Autodesk Fusion 360 part; units mm, degrees
note: some values were not read from the file. Chosen so that the rebuilt part matches the saved one: a direction. Set by a fixed rule: which sketch regions a step uses.
(part 5 of 8)
  spline S19 degree 5 poles (-15.803, -23.1572) (-15.8053, -23.1631) (-15.8097, -23.1748) (-15.8163, -23.1924) (-15.8251, -23.2159) (-15.8359, -23.2453) (-15.8465, -23.2747) (-15.857, -23.304) (-15.8673, -23.3334) (-15.8775, -23.3628) (-15.8876, -23.3922) (-15.8975, -23.4216) (-15.9072, -23.451) (-15.9169, -23.4804) (-15.9263, -23.5098) (-15.9356, -23.5392) (-15.9448, -23.5686) (-15.9538, -23.598) (-15.9626, -23.6275) (-15.9713, -23.6569) (-15.9799, -23.6863) (-15.9882, -23.7157) (-15.9965, -23.7451) (-16.0045, -23.7745) (-16.0124, -23.8039) (-16.0202, -23.8333) (-16.0277, -23.8627) (-16.0352, -23.8921) (-16.0424, -23.9215) (-16.0495, -23.9508) (-16.0564, -23.9802) (-16.0632, -24.0096) (-16.0697, -24.0389) (-16.0761, -24.0683) (-16.0824, -24.0976) (-16.0884, -24.1269) (-16.0943, -24.1562) (-16.1, -24.1855) (-16.1055, -24.2148) (-16.1109, -24.2441) (-16.116, -24.2734) (-16.121, -24.3026) (-16.1258, -24.3319) (-16.1303, -24.3611) (-16.1347, -24.3903) (-16.1389, -24.4195) (-16.1429, -24.4487) (-16.1467, -24.4778) (-16.1503, -24.5069) (-16.1537, -24.536) (-16.1569, -24.5651) (-16.1598, -24.5942) (-16.1625, -24.6232) (-16.165, -24.6522) (-16.1672, -24.6812) (-16.1692, -24.7101) (-16.171, -24.7391) (-16.1726, -24.768) (-16.174, -24.7968) (-16.1751, -24.8257) (-16.1759, -24.8544) (-16.1763, -24.8832) (-16.1764, -24.9118) (-16.1761, -24.9405) (-16.1754, -24.969) (-16.1745, -24.9976) (-16.1735, -25.0261) (-16.1722, -25.0545) (-16.1707, -25.0829) (-16.1687, -25.1112) (-16.1659, -25.1394) (-16.1628, -25.1618) (-16.1599, -25.1785) (-16.1576, -25.1896) (-16.1565, -25.1951) knots -1 -1 -1 -1 -1 -1 -0.98571429 -0.97142857 -0.95714286 -0.94285714 -0.92857143 -0.91428571 -0.9 -0.88571429 -0.87142857 -0.85714286 -0.84285714 -0.82857143 -0.81428571 -0.8 -0.78571429 -0.77142857 -0.75714286 -0.74285714 -0.72857143 -0.71428571 -0.7 -0.68571429 -0.67142857 -0.65714286 -0.64285714 -0.62857143 -0.61428571 -0.6 -0.58571429 -0.57142857 -0.55714286 -0.54285714 -0.52857143 -0.51428571 -0.5 -0.48571429 -0.47142857 -0.45714286 -0.44285714 -0.42857143 -0.41428571 -0.4 -0.38571429 -0.37142857 -0.35714286 -0.34285714 -0.32857143 -0.31428571 -0.3 -0.28571429 -0.27142857 -0.25714286 -0.24285714 -0.22857143 -0.21428571 -0.2 -0.18571429 -0.17142857 -0.15714286 -0.14285714 -0.12857143 -0.11428571 -0.1 -0.08571429 -0.07142857 -0.05714286 -0.04285714 -0.02857143 -0.01428571 0 0 0 0 0 0
  line L19 (-16.1565, -25.1951) -> (-16.0752, -25.5744)
  arc A39 (-16.1513, -25.6929) -> (-16.0752, -25.5744) centre (-16.173, -25.5953) ccw
  arc A40 (-16.1513, -25.6929) -> (-17.1506, -25.9604) centre (-13.5, -37.5997) ccw
  arc A41 (-17.2757, -25.8957) -> (-17.1506, -25.9604) centre (-17.1805, -25.865) ccw
  line L20 (-17.2757, -25.8957) -> (-17.3947, -25.5265)
  spline S20 degree 5 poles (-17.3947, -25.5265) (-17.3965, -25.5211) (-17.4001, -25.5104) (-17.4059, -25.4945) (-17.4144, -25.4735) (-17.426, -25.4477) (-17.4384, -25.4222) (-17.4513, -25.3969) (-17.4645, -25.3716) (-17.4778, -25.3464) (-17.4912, -25.3212) (-17.505, -25.2961) (-17.519, -25.2712) (-17.5334, -25.2464) (-17.5481, -25.2217) (-17.5632, -25.1972) (-17.5785, -25.1727) (-17.5941, -25.1484) (-17.6099, -25.1242) (-17.6259, -25.1) (-17.6421, -25.0759) (-17.6585, -25.052) (-17.6752, -25.0281) (-17.692, -25.0043) (-17.7091, -24.9806) (-17.7263, -24.9569) (-17.7438, -24.9334) (-17.7615, -24.91) (-17.7793, -24.8866) (-17.7974, -24.8634) (-17.8156, -24.8402) (-17.834, -24.817) (-17.8525, -24.794) (-17.8713, -24.7711) (-17.8902, -24.7482) (-17.9093, -24.7254) (-17.9285, -24.7027) (-17.9479, -24.6801) (-17.9675, -24.6576) (-17.9872, -24.6351) (-18.0071, -24.6127) (-18.0272, -24.5904) (-18.0474, -24.5682) (-18.0677, -24.5461) (-18.0883, -24.524) (-18.1089, -24.502) (-18.1297, -24.4801) (-18.1507, -24.4583) (-18.1718, -24.4365) (-18.193, -24.4148) (-18.2144, -24.3932) (-18.236, -24.3717) (-18.2576, -24.3503) (-18.2794, -24.3289) (-18.3014, -24.3076) (-18.3235, -24.2864) (-18.3457, -24.2653) (-18.3681, -24.2442) (-18.3905, -24.2232) (-18.4132, -24.2023) (-18.4359, -24.1815) (-18.4588, -24.1607) (-18.4818, -24.1401) (-18.505, -24.1195) (-18.5282, -24.0989) (-18.5516, -24.0785) (-18.5751, -24.0581) (-18.5988, -24.0378) (-18.6225, -24.0176) (-18.6464, -23.9975) (-18.6704, -23.9774) (-18.6897, -23.9615) (-18.7043, -23.9495) (-18.714, -23.9415) (-18.7189, -23.9376) knots 0 0 0 0 0 0 0.01428571 0.02857143 0.04285714 0.05714286 0.07142857 0.08571429 0.1 0.11428571 0.12857143 0.14285714 0.15714286 0.17142857 0.18571429 0.2 0.21428571 0.22857143 0.24285714 0.25714286 0.27142857 0.28571429 0.3 0.31428571 0.32857143 0.34285714 0.35714286 0.37142857 0.38571429 0.4 0.41428571 0.42857143 0.44285714 0.45714286 0.47142857 0.48571429 0.5 0.51428571 0.52857143 0.54285714 0.55714286 0.57142857 0.58571429 0.6 0.61428571 0.62857143 0.64285714 0.65714286 0.67142857 0.68571429 0.7 0.71428571 0.72857143 0.74285714 0.75714286 0.77142857 0.78571429 0.8 0.81428571 0.82857143 0.84285714 0.85714286 0.87142857 0.88571429 0.9 0.91428571 0.92857143 0.94285714 0.95714286 0.97142857 0.98571429 1 1 1 1 1 1
  arc A42 (-18.7189, -23.9376) -> (-19.4626, -24.2454) centre (-13.5, -37.5997) ccw
  spline S21 degree 5 poles (-19.4626, -24.2454) (-19.4632, -24.2516) (-19.4645, -24.2641) (-19.4663, -24.2828) (-19.4687, -24.3078) (-19.4715, -24.339) (-19.4741, -24.3701) (-19.4767, -24.4012) (-19.4791, -24.4322) (-19.4813, -24.4633) (-19.4834, -24.4943) (-19.4854, -24.5252) (-19.4872, -24.5562) (-19.4888, -24.587) (-19.4904, -24.6179) (-19.4918, -24.6487) (-19.493, -24.6795) (-19.4941, -24.7102) (-19.495, -24.7409) (-19.4958, -24.7716) (-19.4964, -24.8022) (-19.4969, -24.8328) (-19.4972, -24.8633) (-19.4974, -24.8938) (-19.4974, -24.9242) (-19.4973, -24.9546) (-19.497, -24.985) (-19.4966, -25.0153) (-19.496, -25.0456) (-19.4952, -25.0758) (-19.4943, -25.1059) (-19.4932, -25.136) (-19.492, -25.1661) (-19.4906, -25.1961) (-19.489, -25.226) (-19.4873, -25.2559) (-19.4853, -25.2858) (-19.4833, -25.3156) (-19.481, -25.3453) (-19.4786, -25.3749) (-19.476, -25.4045) (-19.4732, -25.4341) (-19.4703, -25.4636) (-19.4671, -25.493) (-19.4638, -25.5223) (-19.4603, -25.5516) (-19.4566, -25.5808) (-19.4527, -25.6099) (-19.4487, -25.639) (-19.4444, -25.668) (-19.4399, -25.6969) (-19.4353, -25.7258) (-19.4304, -25.7545) (-19.4252, -25.7831) (-19.4199, -25.8117) (-19.4143, -25.8402) (-19.4086, -25.8686) (-19.4026, -25.8969) (-19.3965, -25.9252) (-19.3901, -25.9533) (-19.3834, -25.9813) (-19.3764, -26.0092) (-19.369, -26.0369) (-19.3613, -26.0644) (-19.3533, -26.0919) (-19.3451, -26.1192) (-19.3367, -26.1464) (-19.3281, -26.1736) (-19.3193, -26.2006) (-19.31, -26.2275) (-19.3, -26.254) (-19.2912, -26.2748) (-19.2841, -26.2902) (-19.2791, -26.3003) (-19.2765, -26.3053) knots -1 -1 -1 -1 -1 -1 -0.98571429 -0.97142857 -0.95714286 -0.94285714 -0.92857143 -0.91428571 -0.9 -0.88571429 -0.87142857 -0.85714286 -0.84285714 -0.82857143 -0.81428571 -0.8 -0.78571429 -0.77142857 -0.75714286 -0.74285714 -0.72857143 -0.71428571 -0.7 -0.68571429 -0.67142857 -0.65714286 -0.64285714 -0.62857143 -0.61428571 -0.6 -0.58571429 -0.57142857 -0.55714286 -0.54285714 -0.52857143 -0.51428571 -0.5 -0.48571429 -0.47142857 -0.45714286 -0.44285714 -0.42857143 -0.41428571 -0.4 -0.38571429 -0.37142857 -0.35714286 -0.34285714 -0.32857143 -0.31428571 -0.3 -0.28571429 -0.27142857 -0.25714286 -0.24285714 -0.22857143 -0.21428571 -0.2 -0.18571429 -0.17142857 -0.15714286 -0.14285714 -0.12857143 -0.11428571 -0.1 -0.08571429 -0.07142857 -0.05714286 -0.04285714 -0.02857143 -0.01428571 0 0 0 0 0 0
  line L21 (-19.2765, -26.3053) -> (-19.0999, -26.6507)
  arc A43 (-19.1426, -26.7849) -> (-19.0999, -26.6507) centre (-19.1889, -26.6962) ccw
  arc A44 (-19.1426, -26.7849) -> (-20.0387, -27.3018) centre (-13.5, -37.5997) ccw
  arc A45 (-20.1762, -27.2717) -> (-20.0387, -27.3018) centre (-20.0923, -27.2174) ccw
  line L22 (-20.1762, -27.2717) -> (-20.3868, -26.946)
  spline S22 degree 5 poles (-20.3868, -26.946) (-20.3899, -26.9412) (-20.3961, -26.9318) (-20.4059, -26.9179) (-20.4195, -26.8999) (-20.4374, -26.8779) (-20.456, -26.8565) (-20.475, -26.8353) (-20.4942, -26.8143) (-20.5136, -26.7934) (-20.5332, -26.7726) (-20.5529, -26.7519) (-20.5729, -26.7315) (-20.5932, -26.7112) (-20.6138, -26.6912) (-20.6347, -26.6714) (-20.6559, -26.6518) (-20.6772, -26.6323) (-20.6988, -26.613) (-20.7205, -26.5938) (-20.7424, -26.5747) (-20.7644, -26.5558) (-20.7867, -26.537) (-20.8091, -26.5184) (-20.8317, -26.4999) (-20.8545, -26.4816) (-20.8775, -26.4634) (-20.9006, -26.4453) (-20.9239, -26.4274) (-20.9473, -26.4096) (-20.9709, -26.3919) (-20.9947, -26.3743) (-21.0186, -26.3569) (-21.0426, -26.3396) (-21.0668, -26.3224) (-21.0911, -26.3053) (-21.1156, -26.2884) (-21.1402, -26.2715) (-21.1649, -26.2548) (-21.1898, -26.2383) (-21.2148, -26.2218) (-21.24, -26.2054) (-21.2652, -26.1892) (-21.2906, -26.1731) (-21.3162, -26.1571) (-21.3418, -26.1412) (-21.3676, -26.1254) (-21.3935, -26.1097) (-21.4195, -26.0942) (-21.4456, -26.0787) (-21.4719, -26.0634) (-21.4983, -26.0482) (-21.5247, -26.0331) (-21.5513, -26.0181) (-21.578, -26.0032) (-21.6049, -25.9884) (-21.6318, -25.9738) (-21.6588, -25.9592) (-21.686, -25.9448) (-21.7133, -25.9304) (-21.7406, -25.9162) (-21.7681, -25.9021) (-21.7957, -25.8881) (-21.8234, -25.8742) (-21.8511, -25.8604) (-21.879, -25.8467) (-21.907, -25.8331) (-21.9351, -25.8196) (-21.9633, -25.8062) (-21.9916, -25.793) (-22.02, -25.7798) (-22.0428, -25.7694) (-22.0599, -25.7616) (-22.0713, -25.7564) (-22.0771, -25.7538) knots 0 0 0 0 0 0 0.01428571 0.02857143 0.04285714 0.05714286 0.07142857 0.08571429 0.1 0.11428571 0.12857143 0.14285714 0.15714286 0.17142857 0.18571429 0.2 0.21428571 0.22857143 0.24285714 0.25714286 0.27142857 0.28571429 0.3 0.31428571 0.32857143 0.34285714 0.35714286 0.37142857 0.38571429 0.4 0.41428571 0.42857143 0.44285714 0.45714286 0.47142857 0.48571429 0.5 0.51428571 0.52857143 0.54285714 0.55714286 0.57142857 0.58571429 0.6 0.61428571 0.62857143 0.64285714 0.65714286 0.67142857 0.68571429 0.7 0.71428571 0.72857143 0.74285714 0.75714286 0.77142857 0.78571429 0.8 0.81428571 0.82857143 0.84285714 0.85714286 0.87142857 0.88571429 0.9 0.91428571 0.92857143 0.94285714 0.95714286 0.97142857 0.98571429 1 1 1 1 1 1
  arc A46 (-22.0771, -25.7538) -> (-22.7158, -26.2436) centre (-13.5, -37.5997) ccw
  spline S23 degree 5 poles (-22.7158, -26.2436) (-22.7148, -26.2498) (-22.7127, -26.2622) (-22.7097, -26.2808) (-22.7055, -26.3055) (-22.7001, -26.3363) (-22.6947, -26.3671) (-22.689, -26.3978) (-22.6833, -26.4284) (-22.6775, -26.459) (-22.6715, -26.4894) (-22.6653, -26.5199) (-22.6591, -26.5502) (-22.6527, -26.5805) (-22.6462, -26.6107) (-22.6396, -26.6408) (-22.6328, -26.6708) (-22.6259, -26.7008) (-22.6188, -26.7307) (-22.6116, -26.7605) (-22.6043, -26.7903) (-22.5969, -26.8199) (-22.5893, -26.8495) (-22.5816, -26.879) (-22.5737, -26.9084) (-22.5657, -26.9377) (-22.5576, -26.967) (-22.5493, -26.9961) (-22.5409, -27.0252) (-22.5324, -27.0542) (-22.5237, -27.0831) (-22.5148, -27.1119) (-22.5059, -27.1406) (-22.4967, -27.1692) (-22.4875, -27.1977) (-22.478, -27.2262) (-22.4685, -27.2545) (-22.4588, -27.2827) (-22.4489, -27.3108) (-22.4389, -27.3389) (-22.4287, -27.3668) (-22.4184, -27.3946) (-22.4079, -27.4223) (-22.3973, -27.4499) (-22.3865, -27.4774) (-22.3755, -27.5048) (-22.3644, -27.532) (-22.3531, -27.5592) (-22.3416, -27.5862) (-22.33, -27.6131) (-22.3182, -27.6399) (-22.3062, -27.6665) (-22.2941, -27.693) (-22.2817, -27.7194) (-22.2691, -27.7456) (-22.2564, -27.7716) (-22.2435, -27.7976) (-22.2304, -27.8234) (-22.2172, -27.8491) (-22.2037, -27.8746) (-22.19, -27.8999) (-22.176, -27.925) (-22.1617, -27.9499) (-22.1472, -27.9745) (-22.1323, -27.9989) (-22.1173, -28.0232) (-22.1021, -28.0473) (-22.0868, -28.0714) (-22.0713, -28.0952) (-22.0554, -28.1187) (-22.0389, -28.1417) (-22.025, -28.1596) (-22.0141, -28.1726) (-22.0066, -28.181) (-22.0029, -28.1852) knots -1 -1 -1 -1 -1 -1 -0.98571429 -0.97142857 -0.95714286 -0.94285714 -0.92857143 -0.91428571 -0.9 -0.88571429 -0.87142857 -0.85714286 -0.84285714 -0.82857143 -0.81428571 -0.8 -0.78571429 -0.77142857 -0.75714286 -0.74285714 -0.72857143 -0.71428571 -0.7 -0.68571429 -0.67142857 -0.65714286 -0.64285714 -0.62857143 -0.61428571 -0.6 -0.58571429 -0.57142857 -0.55714286 -0.54285714 -0.52857143 -0.51428571 -0.5 -0.48571429 -0.47142857 -0.45714286 -0.44285714 -0.42857143 -0.41428571 -0.4 -0.38571429 -0.37142857 -0.35714286 -0.34285714 -0.32857143 -0.31428571 -0.3 -0.28571429 -0.27142857 -0.25714286 -0.24285714 -0.22857143 -0.21428571 -0.2 -0.18571429 -0.17142857 -0.15714286 -0.14285714 -0.12857143 -0.11428571 -0.1 -0.08571429 -0.07142857 -0.05714286 -0.04285714 -0.02857143 -0.01428571 0 0 0 0 0 0
  line L23 (-22.0029, -28.1852) -> (-21.7429, -28.4731)
  arc A47 (-21.7495, -28.6138) -> (-21.7429, -28.4731) centre (-21.8171, -28.5401) ccw
  arc A48 (-21.7495, -28.6138) -> (-22.4811, -29.3451) centre (-13.5, -37.5997) ccw
  arc A49 (-22.6218, -29.3516) -> (-22.4811, -29.3451) centre (-22.5548, -29.2774) ccw
  line L24 (-22.6218, -29.3516) -> (-22.9095, -29.0914)
  spline S24 degree 5 poles (-22.9095, -29.0914) (-22.9137, -29.0876) (-22.9222, -29.0801) (-22.9352, -29.0692) (-22.953, -29.0553) (-22.976, -29.0388) (-22.9995, -29.0229) (-23.0234, -29.0074) (-23.0474, -28.9921) (-23.0715, -28.9769) (-23.0958, -28.9618) (-23.1202, -28.947) (-23.1448, -28.9324) (-23.1697, -28.9181) (-23.1948, -28.9041) (-23.2201, -28.8904) (-23.2456, -28.8769) (-23.2713, -28.8636) (-23.2971, -28.8505) (-23.323, -28.8376) (-23.3491, -28.8249) (-23.3753, -28.8123) (-23.4016, -28.7999) (-23.4281, -28.7877) (-23.4547, -28.7757) (-23.4815, -28.7639) (-23.5084, -28.7523) (-23.5354, -28.7408) (-23.5626, -28.7295) (-23.5898, -28.7184) (-23.6172, -28.7074) (-23.6446, -28.6966) (-23.6722, -28.6859) (-23.6999, -28.6754) (-23.7277, -28.6651) (-23.7557, -28.6549) (-23.7837, -28.6449) (-23.8118, -28.635) (-23.84, -28.6252) (-23.8684, -28.6157) (-23.8968, -28.6062) (-23.9253, -28.5969) (-23.9539, -28.5878) (-23.9826, -28.5788) (-24.0114, -28.5699) (-24.0403, -28.5612) (-24.0693, -28.5527) (-24.0983, -28.5442) (-24.1275, -28.5359) (-24.1567, -28.5278) (-24.1861, -28.5198) (-24.2155, -28.5119) (-24.245, -28.5042) (-24.2745, -28.4966) (-24.3042, -28.4891) (-24.3339, -28.4818) (-24.3637, -28.4746) (-24.3936, -28.4675) (-24.4236, -28.4606) (-24.4536, -28.4538) (-24.4837, -28.4472) (-24.5139, -28.4406) (-24.5442, -28.4342) (-24.5745, -28.428) (-24.605, -28.4218) (-24.6354, -28.4158) (-24.666, -28.4099) (-24.6966, -28.4042) (-24.7273, -28.3986) (-24.758, -28.3931) (-24.7889, -28.3877) (-24.8136, -28.3835) (-24.8321, -28.3804) (-24.8445, -28.3784) (-24.8507, -28.3774) knots 0 0 0 0 0 0 0.01428571 0.02857143 0.04285714 0.05714286 0.07142857 0.08571429 0.1 0.11428571 0.12857143 0.14285714 0.15714286 0.17142857 0.18571429 0.2 0.21428571 0.22857143 0.24285714 0.25714286 0.27142857 0.28571429 0.3 0.31428571 0.32857143 0.34285714 0.35714286 0.37142857 0.38571429 0.4 0.41428571 0.42857143 0.44285714 0.45714286 0.47142857 0.48571429 0.5 0.51428571 0.52857143 0.54285714 0.55714286 0.57142857 0.58571429 0.6 0.61428571 0.62857143 0.64285714 0.65714286 0.67142857 0.68571429 0.7 0.71428571 0.72857143 0.74285714 0.75714286 0.77142857 0.78571429 0.8 0.81428571 0.82857143 0.84285714 0.85714286 0.87142857 0.88571429 0.9 0.91428571 0.92857143 0.94285714 0.95714286 0.97142857 0.98571429 1 1 1 1 1 1
  arc A50 (-24.8507, -28.3774) -> (-25.3409, -29.0158) centre (-13.5, -37.5997) ccw
  spline S25 degree 5 poles (-25.3409, -29.0158) (-25.3383, -29.0215) (-25.3332, -29.033) (-25.3254, -29.0501) (-25.315, -29.0729) (-25.3018, -29.1013) (-25.2886, -29.1296) (-25.2752, -29.1578) (-25.2617, -29.1859) (-25.2482, -29.2139) (-25.2345, -29.2418) (-25.2207, -29.2696) (-25.2068, -29.2973) (-25.1928, -29.3248) (-25.1787, -29.3523) (-25.1645, -29.3797) (-25.1502, -29.407) (-25.1358, -29.4341) (-25.1212, -29.4612) (-25.1066, -29.4881) (-25.0918, -29.515) (-25.0769, -29.5417) (-25.062, -29.5683) (-25.0469, -29.5948) (-25.0317, -29.6211) (-25.0164, -29.6474) (-25.0009, -29.6736) (-24.9854, -29.6996) (-24.9698, -29.7255) (-24.954, -29.7513) (-24.9381, -29.7769) (-24.9221, -29.8025) (-24.906, -29.8279) (-24.8898, -29.8531) (-24.8735, -29.8783) (-24.857, -29.9033) (-24.8404, -29.9282) (-24.8237, -29.953) (-24.8069, -29.9776) (-24.79, -30.0021) (-24.773, -30.0264) (-24.7558, -30.0506) (-24.7385, -30.0746) (-24.7211, -30.0985) (-24.7035, -30.1223) (-24.6858, -30.1459) (-24.668, -30.1693) (-24.6501, -30.1926) (-24.632, -30.2158) (-24.6139, -30.2388) (-24.5955, -30.2616) (-24.5771, -30.2842) (-24.5585, -30.3066) (-24.5397, -30.3289) (-24.5208, -30.351) (-24.5017, -30.3728) (-24.4825, -30.3946) (-24.4632, -30.4161) (-24.4438, -30.4375) (-24.4242, -30.4587) (-24.4044, -30.4796) (-24.3844, -30.5002) (-24.3642, -30.5205) (-24.3437, -30.5405) (-24.323, -30.5603) (-24.3022, -30.5798) (-24.2813, -30.5992) (-24.2603, -30.6185) (-24.2392, -30.6375) (-24.2178, -30.6561) (-24.1959, -30.674) (-24.1778, -30.6877) (-24.1639, -30.6974) (-24.1545, -30.7037) (-24.1498, -30.7067) knots -1 -1 -1 -1 -1 -1 -0.98571429 -0.97142857 -0.95714286 -0.94285714 -0.92857143 -0.91428571 -0.9 -0.88571429 -0.87142857 -0.85714286 -0.84285714 -0.82857143 -0.81428571 -0.8 -0.78571429 -0.77142857 -0.75714286 -0.74285714 -0.72857143 -0.71428571 -0.7 -0.68571429 -0.67142857 -0.65714286 -0.64285714 -0.62857143 -0.61428571 -0.6 -0.58571429 -0.57142857 -0.55714286 -0.54285714 -0.52857143 -0.51428571 -0.5 -0.48571429 -0.47142857 -0.45714286 -0.44285714 -0.42857143 -0.41428571 -0.4 -0.38571429 -0.37142857 -0.35714286 -0.34285714 -0.32857143 -0.31428571 -0.3 -0.28571429 -0.27142857 -0.25714286 -0.24285714 -0.22857143 -0.21428571 -0.2 -0.18571429 -0.17142857 -0.15714286 -0.14285714 -0.12857143 -0.11428571 -0.1 -0.08571429 -0.07142857 -0.05714286 -0.04285714 -0.02857143 -0.01428571 0 0 0 0 0 0
  line L25 (-24.1498, -30.7067) -> (-23.8241, -30.9175)
  arc A51 (-23.7941, -31.0551) -> (-23.8241, -30.9175) centre (-23.8785, -31.0014) ccw
  arc A52 (-23.7941, -31.0551) -> (-24.3116, -31.9508) centre (-13.5, -37.5997) ccw
  arc A53 (-24.4458, -31.9935) -> (-24.3116, -31.9508) centre (-24.4002, -31.9045) ccw
  line L26 (-24.4458, -31.9935) -> (-24.791, -31.8167)
  spline S26 degree 5 poles (-24.791, -31.8167) (-24.7961, -31.8141) (-24.8062, -31.8091) (-24.8216, -31.8019) (-24.8424, -31.7931) (-24.8689, -31.7831) (-24.8957, -31.7738) (-24.9227, -31.765) (-24.9499, -31.7564) (-24.9771, -31.748) (-25.0045, -31.7397) (-25.0319, -31.7317) (-25.0594, -31.724) (-25.0871, -31.7166) (-25.115, -31.7096) (-25.143, -31.7029) (-25.1711, -31.6965) (-25.1994, -31.6903) (-25.2277, -31.6843) (-25.2561, -31.6786) (-25.2846, -31.673) (-25.3131, -31.6676) (-25.3418, -31.6625) (-25.3705, -31.6576) (-25.3993, -31.6529) (-25.4283, -31.6484) (-25.4573, -31.6441) (-25.4863, -31.64) (-25.5155, -31.6361) (-25.5447, -31.6324) (-25.5739, -31.6289) (-25.6033, -31.6256) (-25.6327, -31.6224) (-25.6622, -31.6194) (-25.6917, -31.6166) (-25.7213, -31.614) (-25.751, -31.6116) (-25.7807, -31.6093) (-25.8105, -31.6072) (-25.8403, -31.6053) (-25.8702, -31.6036) (-25.9002, -31.602) (-25.9302, -31.6005) (-25.9602, -31.5993) (-25.9903, -31.5982) (-26.0205, -31.5972) (-26.0507, -31.5965) (-26.0809, -31.5958) (-26.1112, -31.5954) (-26.1416, -31.5951) (-26.172, -31.5949) (-26.2024, -31.5949) (-26.2329, -31.5951) (-26.2635, -31.5954) (-26.294, -31.5959) (-26.3247, -31.5965) (-26.3553, -31.5973) (-26.386, -31.5982) (-26.4167, -31.5992) (-26.4475, -31.6005) (-26.4783, -31.6018) (-26.5092, -31.6033) (-26.5401, -31.605) (-26.571, -31.6068) (-26.602, -31.6087) (-26.633, -31.6108) (-26.664, -31.613) (-26.6951, -31.6154) (-26.7262, -31.6179) (-26.7573, -31.6206) (-26.7885, -31.6234) (-26.8134, -31.6257) (-26.8321, -31.6275) (-26.8446, -31.6288) (-26.8509, -31.6294) knots 0 0 0 0 0 0 0.01428571 0.02857143 0.04285714 0.05714286 0.07142857 0.08571429 0.1 0.11428571 0.12857143 0.14285714 0.15714286 0.17142857 0.18571429 0.2 0.21428571 0.22857143 0.24285714 0.25714286 0.27142857 0.28571429 0.3 0.31428571 0.32857143 0.34285714 0.35714286 0.37142857 0.38571429 0.4 0.41428571 0.42857143 0.44285714 0.45714286 0.47142857 0.48571429 0.5 0.51428571 0.52857143 0.54285714 0.55714286 0.57142857 0.58571429 0.6 0.61428571 0.62857143 0.64285714 0.65714286 0.67142857 0.68571429 0.7 0.71428571 0.72857143 0.74285714 0.75714286 0.77142857 0.78571429 0.8 0.81428571 0.82857143 0.84285714 0.85714286 0.87142857 0.88571429 0.9 0.91428571 0.92857143 0.94285714 0.95714286 0.97142857 0.98571429 1 1 1 1 1 1
  arc A54 (-26.8509, -31.6294) -> (-27.1591, -32.3729) centre (-13.5, -37.5997) ccw
  spline S27 degree 5 poles (-27.1591, -32.3729) (-27.1551, -32.3778) (-27.1472, -32.3875) (-27.1353, -32.4021) (-27.1193, -32.4214) (-27.0992, -32.4454) (-27.0791, -32.4693) (-27.0589, -32.4931) (-27.0386, -32.5167) (-27.0183, -32.5403) (-26.9979, -32.5637) (-26.9773, -32.587) (-26.9568, -32.6101) (-26.9361, -32.6331) (-26.9154, -32.656) (-26.8945, -32.6788) (-26.8737, -32.7014) (-26.8527, -32.7239) (-26.8316, -32.7463) (-26.8105, -32.7685) (-26.7893, -32.7906) (-26.768, -32.8126) (-26.7467, -32.8344) (-26.7253, -32.8561) (-26.7037, -32.8776) (-26.6822, -32.899) (-26.6605, -32.9203) (-26.6388, -32.9414) (-26.6169, -32.9624) (-26.595, -32.9832) (-26.5731, -33.0039) (-26.551, -33.0244) (-26.5289, -33.0448) (-26.5067, -33.065) (-26.4844, -33.0851) (-26.462, -33.105) (-26.4395, -33.1247) (-26.417, -33.1443) (-26.3944, -33.1637) (-26.3717, -33.183) (-26.349, -33.2021) (-26.3261, -33.221) (-26.3032, -33.2398) (-26.2802, -33.2584) (-26.2571, -33.2768) (-26.2339, -33.295) (-26.2106, -33.313) (-26.1873, -33.3309) (-26.1638, -33.3486) (-26.1403, -33.3661) (-26.1167, -33.3833) (-26.093, -33.4004) (-26.0692, -33.4173) (-26.0453, -33.4339) (-26.0214, -33.4503) (-25.9973, -33.4665) (-25.9732, -33.4826) (-25.9489, -33.4984) (-25.9246, -33.514) (-25.9002, -33.5294) (-25.8757, -33.5445) (-25.851, -33.5592) (-25.8262, -33.5736) (-25.8013, -33.5876) (-25.7762, -33.6014) (-25.751, -33.6148) (-25.7258, -33.6282) (-25.7006, -33.6413) (-25.6752, -33.6542) (-25.6497, -33.6666) (-25.6239, -33.6783) (-25.603, -33.6868) (-25.587, -33.6926) (-25.5763, -33.6962) (-25.5709, -33.698) knots -1 -1 -1 -1 -1 -1 -0.98571429 -0.97142857 -0.95714286 -0.94285714 -0.92857143 -0.91428571 -0.9 -0.88571429 -0.87142857 -0.85714286 -0.84285714 -0.82857143 -0.81428571 -0.8 -0.78571429 -0.77142857 -0.75714286 -0.74285714 -0.72857143 -0.71428571 -0.7 -0.68571429 -0.67142857 -0.65714286 -0.64285714 -0.62857143 -0.61428571 -0.6 -0.58571429 -0.57142857 -0.55714286 -0.54285714 -0.52857143 -0.51428571 -0.5 -0.48571429 -0.47142857 -0.45714286 -0.44285714 -0.42857143 -0.41428571 -0.4 -0.38571429 -0.37142857 -0.35714286 -0.34285714 -0.32857143 -0.31428571 -0.3 -0.28571429 -0.27142857 -0.25714286 -0.24285714 -0.22857143 -0.21428571 -0.2 -0.18571429 -0.17142857 -0.15714286 -0.14285714 -0.12857143 -0.11428571 -0.1 -0.08571429 -0.07142857 -0.05714286 -0.04285714 -0.02857143 -0.01428571 0 0 0 0 0 0
  line L27 (-25.5709, -33.698) -> (-25.2018, -33.8173)
  arc A55 (-25.1372, -33.9424) -> (-25.2018, -33.8173) centre (-25.2326, -33.9124) ccw
  arc A56 (-25.1372, -33.9424) -> (-25.4052, -34.9415) centre (-13.5, -37.5997) ccw
  arc A57 (-25.5238, -35.0175) -> (-25.4052, -34.9415) centre (-25.5028, -34.9197) ccw
  line L28 (-25.5238, -35.0175) -> (-25.9031, -34.9361)
  spline S28 degree 5 poles (-25.9031, -34.9361) (-25.9086, -34.9349) (-25.9197, -34.9327) (-25.9364, -34.9297) (-25.9588, -34.9266) (-25.9869, -34.9238) (-26.0153, -34.9218) (-26.0437, -34.9202) (-26.0721, -34.919) (-26.1006, -34.9179) (-26.1291, -34.917) (-26.1577, -34.9163) (-26.1863, -34.916) (-26.215, -34.916) (-26.2437, -34.9164) (-26.2725, -34.9172) (-26.3013, -34.9183) (-26.3302, -34.9197) (-26.3591, -34.9212) (-26.388, -34.923) (-26.417, -34.925) (-26.4459, -34.9272) (-26.4749, -34.9297) (-26.504, -34.9324) (-26.533, -34.9353) (-26.5621, -34.9384) (-26.5912, -34.9418) (-26.6204, -34.9454) (-26.6495, -34.9492) (-26.6787, -34.9532) (-26.7079, -34.9573) (-26.7371, -34.9617) (-26.7663, -34.9663) (-26.7956, -34.971) (-26.8248, -34.976) (-26.8541, -34.9811) (-26.8834, -34.9864) (-26.9127, -34.9919) (-26.942, -34.9976) (-26.9713, -35.0035) (-27.0006, -35.0095) (-27.03, -35.0157) (-27.0593, -35.0221) (-27.0887, -35.0287) (-27.118, -35.0354) (-27.1474, -35.0423) (-27.1768, -35.0494) (-27.2062, -35.0566) (-27.2356, -35.064) (-27.265, -35.0716) (-27.2944, -35.0793) (-27.3238, -35.0872) (-27.3532, -35.0952) (-27.3826, -35.1034) (-27.412, -35.1118) (-27.4414, -35.1203) (-27.4708, -35.129) (-27.5002, -35.1378) (-27.5297, -35.1468) (-27.5591, -35.1559) (-27.5885, -35.1652) (-27.6179, -35.1747) (-27.6473, -35.1843) (-27.6767, -35.194) (-27.7061, -35.2039) (-27.7355, -35.2139) (-27.7649, -35.2241) (-27.7943, -35.2344) (-27.8237, -35.2449) (-27.8531, -35.2555) (-27.8825, -35.2663) (-27.906, -35.275) (-27.9236, -35.2816) (-27.9353, -35.2861) (-27.9412, -35.2883) knots 0 0 0 0 0 0 0.01428571 0.02857143 0.04285714 0.05714286 0.07142857 0.08571429 0.1 0.11428571 0.12857143 0.14285714 0.15714286 0.17142857 0.18571429 0.2 0.21428571 0.22857143 0.24285714 0.25714286 0.27142857 0.28571429 0.3 0.31428571 0.32857143 0.34285714 0.35714286 0.37142857 0.38571429 0.4 0.41428571 0.42857143 0.44285714 0.45714286 0.47142857 0.48571429 0.5 0.51428571 0.52857143 0.54285714 0.55714286 0.57142857 0.58571429 0.6 0.61428571 0.62857143 0.64285714 0.65714286 0.67142857 0.68571429 0.7 0.71428571 0.72857143 0.74285714 0.75714286 0.77142857 0.78571429 0.8 0.81428571 0.82857143 0.84285714 0.85714286 0.87142857 0.88571429 0.9 0.91428571 0.92857143 0.94285714 0.95714286 0.97142857 0.98571429 1 1 1 1 1 1
  arc A58 (-27.9412, -35.2883) -> (-28.0465, -36.0863) centre (-13.5, -37.5997) ccw
  spline S29 degree 5 poles (-28.0465, -36.0863) (-28.0414, -36.09) (-28.0312, -36.0973) (-28.0159, -36.1082) (-27.9955, -36.1228) (-27.9699, -36.1408) (-27.9443, -36.1587) (-27.9186, -36.1764) (-27.8929, -36.194) (-27.8671, -36.2115) (-27.8413, -36.2288) (-27.8155, -36.246) (-27.7896, -36.263) (-27.7637, -36.2799) (-27.7378, -36.2966) (-27.7118, -36.3132) (-27.6857, -36.3297) (-27.6597, -36.346) (-27.6335, -36.3621) (-27.6074, -36.3782) (-27.5812, -36.394) (-27.5549, -36.4097) (-27.5287, -36.4253) (-27.5024, -36.4407) (-27.476, -36.4559) (-27.4496, -36.471) (-27.4232, -36.4859) (-27.3967, -36.5007) (-27.3702, -36.5153) (-27.3437, -36.5298) (-27.3171, -36.544) (-27.2905, -36.5582) (-27.2638, -36.5721) (-27.2371, -36.5859) (-27.2104, -36.5995) (-27.1837, -36.6129) (-27.1569, -36.6262) (-27.13, -36.6393) (-27.1032, -36.6522) (-27.0763, -36.6649) (-27.0493, -36.6775) (-27.0224, -36.6899) (-26.9953, -36.702) (-26.9683, -36.714) (-26.9412, -36.7258) (-26.9141, -36.7374) (-26.887, -36.7488) (-26.8598, -36.76) (-26.8326, -36.7711) (-26.8054, -36.7819) (-26.7781, -36.7925) (-26.7508, -36.8028) (-26.7234, -36.8129) (-26.6961, -36.8228) (-26.6687, -36.8325) (-26.6412, -36.8419) (-26.6137, -36.8511) (-26.5862, -36.8602) (-26.5587, -36.869) (-26.5312, -36.8775) (-26.5036, -36.8857) (-26.4759, -36.8936) (-26.4482, -36.901) (-26.4205, -36.9081) (-26.3927, -36.9149) (-26.365, -36.9214) (-26.3372, -36.9278) (-26.3094, -36.9339) (-26.2815, -36.9398) (-26.2537, -36.9452) (-26.2257, -36.9498) (-26.2033, -36.9526) (-26.1864, -36.9541) (-26.1751, -36.9548) (-26.1695, -36.9551) knots -1 -1 -1 -1 -1 -1 -0.98571429 -0.97142857 -0.95714286 -0.94285714 -0.92857143 -0.91428571 -0.9 -0.88571429 -0.87142857 -0.85714286 -0.84285714 -0.82857143 -0.81428571 -0.8 -0.78571429 -0.77142857 -0.75714286 -0.74285714 -0.72857143 -0.71428571 -0.7 -0.68571429 -0.67142857 -0.65714286 -0.64285714 -0.62857143 -0.61428571 -0.6 -0.58571429 -0.57142857 -0.55714286 -0.54285714 -0.52857143 -0.51428571 -0.5 -0.48571429 -0.47142857 -0.45714286 -0.44285714 -0.42857143 -0.41428571 -0.4 -0.38571429 -0.37142857 -0.35714286 -0.34285714 -0.32857143 -0.31428571 -0.3 -0.28571429 -0.27142857 -0.25714286 -0.24285714 -0.22857143 -0.21428571 -0.2 -0.18571429 -0.17142857 -0.15714286 -0.14285714 -0.12857143 -0.11428571 -0.1 -0.08571429 -0.07142857 -0.05714286 -0.04285714 -0.02857143 -0.01428571 0 0 0 0 0 0
  line L29 (-26.1695, -36.9551) -> (-25.7821, -36.9748)
  arc A59 (-25.6873, -37.079) -> (-25.7821, -36.9748) centre (-25.7872, -37.0747) ccw
  arc A60 (-25.6873, -37.079) -> (-25.6876, -38.1134) centre (-13.5, -37.5997) ccw
  arc A61 (-25.7824, -38.2175) -> (-25.6876, -38.1134) centre (-25.7875, -38.1176) ccw
  line L30 (-25.7824, -38.2175) -> (-26.1698, -38.237)
  spline S30 degree 5 poles (-26.1698, -38.237) (-26.1755, -38.2373) (-26.1868, -38.238) (-26.2037, -38.2395) (-26.2261, -38.2422) (-26.254, -38.2468) (-26.2819, -38.2522) (-26.3097, -38.2581) (-26.3375, -38.2642) (-26.3653, -38.2705) (-26.3931, -38.2771) (-26.4209, -38.2838) (-26.4486, -38.2909) (-26.4763, -38.2984) (-26.504, -38.3062) (-26.5316, -38.3144) (-26.5591, -38.3229) (-26.5867, -38.3317) (-26.6142, -38.3407) (-26.6416, -38.3499) (-26.6691, -38.3593) (-26.6965, -38.369) (-26.7239, -38.3788) (-26.7512, -38.3889) (-26.7786, -38.3993) (-26.8058, -38.4098) (-26.8331, -38.4206) (-26.8603, -38.4316) (-26.8875, -38.4428) (-26.9146, -38.4542) (-26.9417, -38.4658) (-26.9688, -38.4776) (-26.9959, -38.4896) (-27.0229, -38.5017) (-27.0499, -38.5141) (-27.0768, -38.5266) (-27.1037, -38.5393) (-27.1306, -38.5522) (-27.1574, -38.5653) (-27.1842, -38.5786) (-27.211, -38.592) (-27.2377, -38.6056) (-27.2644, -38.6194) (-27.2911, -38.6333) (-27.3177, -38.6474) (-27.3443, -38.6617) (-27.3708, -38.6761) (-27.3974, -38.6907) (-27.4238, -38.7054) (-27.4503, -38.7204) (-27.4767, -38.7354) (-27.503, -38.7507) (-27.5293, -38.766) (-27.5556, -38.7816) (-27.5819, -38.7973) (-27.6081, -38.8131) (-27.6343, -38.8291) (-27.6604, -38.8452) (-27.6865, -38.8615) (-27.7125, -38.878) (-27.7385, -38.8946) (-27.7645, -38.9113) (-27.7904, -38.9282) (-27.8163, -38.9452) (-27.8421, -38.9623) (-27.8679, -38.9797) (-27.8937, -38.9971) (-27.9194, -39.0147) (-27.9451, -39.0324) (-27.9707, -39.0503) (-27.9963, -39.0683) (-28.0168, -39.0828) (-28.0321, -39.0937) (-28.0423, -39.1011) (-28.0474, -39.1047) knots 0 0 0 0 0 0 0.01428571 0.02857143 0.04285714 0.05714286 0.07142857 0.08571429 0.1 0.11428571 0.12857143 0.14285714 0.15714286 0.17142857 0.18571429 0.2 0.21428571 0.22857143 0.24285714 0.25714286 0.27142857 0.28571429 0.3 0.31428571 0.32857143 0.34285714 0.35714286 0.37142857 0.38571429 0.4 0.41428571 0.42857143 0.44285714 0.45714286 0.47142857 0.48571429 0.5 0.51428571 0.52857143 0.54285714 0.55714286 0.57142857 0.58571429 0.6 0.61428571 0.62857143 0.64285714 0.65714286 0.67142857 0.68571429 0.7 0.71428571 0.72857143 0.74285714 0.75714286 0.77142857 0.78571429 0.8 0.81428571 0.82857143 0.84285714 0.85714286 0.87142857 0.88571429 0.9 0.91428571 0.92857143 0.94285714 0.95714286 0.97142857 0.98571429 1 1 1 1 1 1
  arc A62 (-28.0474, -39.1047) -> (-27.9425, -39.9028) centre (-13.5, -37.5997) ccw
  spline S31 degree 5 poles (-27.9425, -39.9028) (-27.9367, -39.905) (-27.9249, -39.9094) (-27.9073, -39.916) (-27.8838, -39.9248) (-27.8544, -39.9356) (-27.8251, -39.9462) (-27.7957, -39.9567) (-27.7663, -39.967) (-27.7369, -39.9772) (-27.7075, -39.9873) (-27.6781, -39.9972) (-27.6487, -40.007) (-27.6193, -40.0166) (-27.5899, -40.026) (-27.5605, -40.0353) (-27.5311, -40.0445) (-27.5017, -40.0535) (-27.4723, -40.0623) (-27.4428, -40.071) (-27.4134, -40.0796) (-27.384, -40.088) (-27.3546, -40.0962) (-27.3252, -40.1042) (-27.2958, -40.1121) (-27.2664, -40.1199) (-27.237, -40.1275) (-27.2076, -40.1349) (-27.1783, -40.1421) (-27.1489, -40.1492) (-27.1195, -40.1561) (-27.0902, -40.1629) (-27.0608, -40.1695) (-27.0315, -40.1759) (-27.0021, -40.1821) (-26.9728, -40.1881) (-26.9435, -40.194) (-26.9142, -40.1997) (-26.8849, -40.2053) (-26.8556, -40.2106) (-26.8263, -40.2157) (-26.7971, -40.2207) (-26.7678, -40.2255) (-26.7386, -40.2301) (-26.7094, -40.2344) (-26.6802, -40.2386) (-26.6511, -40.2426) (-26.6219, -40.2464) (-26.5928, -40.25) (-26.5637, -40.2534) (-26.5346, -40.2566) (-26.5055, -40.2595) (-26.4765, -40.2622) (-26.4475, -40.2647) (-26.4185, -40.2669) (-26.3896, -40.2689) (-26.3606, -40.2707) (-26.3318, -40.2723) (-26.3029, -40.2737) (-26.2741, -40.2748) (-26.2453, -40.2756) (-26.2165, -40.276) (-26.1879, -40.2761) (-26.1592, -40.2758) (-26.1307, -40.2751) (-26.1021, -40.2742) (-26.0737, -40.2732) (-26.0452, -40.2719) (-26.0168, -40.2704) (-25.9885, -40.2684) (-25.9603, -40.2656) (-25.9379, -40.2625) (-25.9212, -40.2596) (-25.9101, -40.2574) (-25.9046, -40.2562) knots -1 -1 -1 -1 -1 -1 -0.98571429 -0.97142857 -0.95714286 -0.94285714 -0.92857143 -0.91428571 -0.9 -0.88571429 -0.87142857 -0.85714286 -0.84285714 -0.82857143 -0.81428571 -0.8 -0.78571429 -0.77142857 -0.75714286 -0.74285714 -0.72857143 -0.71428571 -0.7 -0.68571429 -0.67142857 -0.65714286 -0.64285714 -0.62857143 -0.61428571 -0.6 -0.58571429 -0.57142857 -0.55714286 -0.54285714 -0.52857143 -0.51428571 -0.5 -0.48571429 -0.47142857 -0.45714286 -0.44285714 -0.42857143 -0.41428571 -0.4 -0.38571429 -0.37142857 -0.35714286 -0.34285714 -0.32857143 -0.31428571 -0.3 -0.28571429 -0.27142857 -0.25714286 -0.24285714 -0.22857143 -0.21428571 -0.2 -0.18571429 -0.17142857 -0.15714286 -0.14285714 -0.12857143 -0.11428571 -0.1 -0.08571429 -0.07142857 -0.05714286 -0.04285714 -0.02857143 -0.01428571 0 0 0 0 0 0
  line L31 (-25.9046, -40.2562) -> (-25.5253, -40.1749)
  arc A63 (-25.4068, -40.251) -> (-25.5253, -40.1749) centre (-25.5044, -40.2727) ccw
  arc A64 (-25.4068, -40.251) -> (-25.1393, -41.2503) centre (-13.5, -37.5997) ccw
  arc A65 (-25.204, -41.3754) -> (-25.1393, -41.2503) centre (-25.2347, -41.2802) ccw
  line L32 (-25.204, -41.3754) -> (-25.5732, -41.4945)
  spline S32 degree 5 poles (-25.5732, -41.4945) (-25.5786, -41.4962) (-25.5893, -41.4998) (-25.6052, -41.5056) (-25.6262, -41.5141) (-25.652, -41.5258) (-25.6775, -41.5382) (-25.7029, -41.551) (-25.7281, -41.5642) (-25.7534, -41.5775) (-25.7785, -41.591) (-25.8036, -41.6047) (-25.8285, -41.6187) (-25.8533, -41.6331) (-25.878, -41.6478) (-25.9026, -41.6629) (-25.927, -41.6782) (-25.9513, -41.6938) (-25.9755, -41.7096) (-25.9997, -41.7256) (-26.0238, -41.7418) (-26.0478, -41.7582) (-26.0717, -41.7749) (-26.0955, -41.7917) (-26.1192, -41.8088) (-26.1428, -41.826) (-26.1663, -41.8435) (-26.1897, -41.8612) (-26.2131, -41.879) (-26.2364, -41.8971) (-26.2596, -41.9153) (-26.2827, -41.9337) (-26.3057, -41.9522) (-26.3286, -41.971) (-26.3515, -41.9899) (-26.3743, -42.009) (-26.397, -42.0282) (-26.4196, -42.0476) (-26.4421, -42.0672) (-26.4646, -42.087) (-26.487, -42.1068) (-26.5093, -42.1269) (-26.5315, -42.1471) (-26.5537, -42.1675) (-26.5757, -42.188) (-26.5977, -42.2086) (-26.6196, -42.2295) (-26.6414, -42.2504) (-26.6632, -42.2715) (-26.6849, -42.2928) (-26.7065, -42.3142) (-26.728, -42.3357) (-26.7494, -42.3574) (-26.7708, -42.3792) (-26.7921, -42.4011) (-26.8133, -42.4232) (-26.8345, -42.4454) (-26.8555, -42.4678) (-26.8765, -42.4903) (-26.8974, -42.5129) (-26.9182, -42.5356) (-26.939, -42.5585) (-26.9597, -42.5815) (-26.9802, -42.6047) (-27.0008, -42.6279) (-27.0212, -42.6513) (-27.0416, -42.6748) (-27.0619, -42.6985) (-27.0821, -42.7223) (-27.1022, -42.7461) (-27.1223, -42.7702) (-27.1383, -42.7895) (-27.1502, -42.804) (-27.1582, -42.8137) (-27.1621, -42.8186) knots 0 0 0 0 0 0 0.01428571 0.02857143 0.04285714 0.05714286 0.07142857 0.08571429 0.1 0.11428571 0.12857143 0.14285714 0.15714286 0.17142857 0.18571429 0.2 0.21428571 0.22857143 0.24285714 0.25714286 0.27142857 0.28571429 0.3 0.31428571 0.32857143 0.34285714 0.35714286 0.37142857 0.38571429 0.4 0.41428571 0.42857143 0.44285714 0.45714286 0.47142857 0.48571429 0.5 0.51428571 0.52857143 0.54285714 0.55714286 0.57142857 0.58571429 0.6 0.61428571 0.62857143 0.64285714 0.65714286 0.67142857 0.68571429 0.7 0.71428571 0.72857143 0.74285714 0.75714286 0.77142857 0.78571429 0.8 0.81428571 0.82857143 0.84285714 0.85714286 0.87142857 0.88571429 0.9 0.91428571 0.92857143 0.94285714 0.95714286 0.97142857 0.98571429 1 1 1 1 1 1
  arc A66 (-27.1621, -42.8186) -> (-26.8543, -43.5623) centre (-13.5, -37.5997) ccw
  spline S33 degree 5 poles (-26.8543, -43.5623) (-26.8481, -43.5629) (-26.8356, -43.5642) (-26.8169, -43.566) (-26.7919, -43.5684) (-26.7608, -43.5712) (-26.7296, -43.5739) (-26.6985, -43.5764) (-26.6675, -43.5788) (-26.6364, -43.581) (-26.6054, -43.5831) (-26.5745, -43.5851) (-26.5436, -43.5869) (-26.5127, -43.5886) (-26.4818, -43.5901) (-26.451, -43.5915) (-26.4202, -43.5927) (-26.3895, -43.5938) (-26.3588, -43.5947) (-26.3281, -43.5955) (-26.2975, -43.5961) (-26.2669, -43.5966) (-26.2364, -43.597) (-26.2059, -43.5971) (-26.1755, -43.5972) (-26.1451, -43.597) (-26.1147, -43.5967) (-26.0844, -43.5963) (-26.0542, -43.5957) (-26.024, -43.5949) (-25.9938, -43.594) (-25.9637, -43.5929) (-25.9336, -43.5917) (-25.9036, -43.5903) (-25.8737, -43.5887) (-25.8438, -43.587) (-25.8139, -43.5851) (-25.7842, -43.583) (-25.7544, -43.5807) (-25.7248, -43.5783) (-25.6952, -43.5757) (-25.6656, -43.5729) (-25.6361, -43.57) (-25.6067, -43.5668) (-25.5774, -43.5635) (-25.5481, -43.56) (-25.5189, -43.5563) (-25.4898, -43.5524) (-25.4607, -43.5484) (-25.4317, -43.5441) (-25.4028, -43.5397) (-25.374, -43.535) (-25.3452, -43.5301) (-25.3166, -43.5249) (-25.288, -43.5196) (-25.2595, -43.5141) (-25.2311, -43.5083) (-25.2028, -43.5024) (-25.1746, -43.4962) (-25.1464, -43.4898) (-25.1184, -43.4831) (-25.0906, -43.4761) (-25.0628, -43.4688) (-25.0353, -43.461) (-25.0078, -43.453) (-24.9805, -43.4448) (-24.9533, -43.4364) (-24.9261, -43.4278) (-24.8991, -43.419) (-24.8722, -43.4097) (-24.8458, -43.3997) (-24.8249, -43.3909) (-24.8096, -43.3838) (-24.7994, -43.3788) (-24.7944, -43.3762) knots -1 -1 -1 -1 -1 -1 -0.98571429 -0.97142857 -0.95714286 -0.94285714 -0.92857143 -0.91428571 -0.9 -0.88571429 -0.87142857 -0.85714286 -0.84285714 -0.82857143 -0.81428571 -0.8 -0.78571429 -0.77142857 -0.75714286 -0.74285714 -0.72857143 -0.71428571 -0.7 -0.68571429 -0.67142857 -0.65714286 -0.64285714 -0.62857143 -0.61428571 -0.6 -0.58571429 -0.57142857 -0.55714286 -0.54285714 -0.52857143 -0.51428571 -0.5 -0.48571429 -0.47142857 -0.45714286 -0.44285714 -0.42857143 -0.41428571 -0.4 -0.38571429 -0.37142857 -0.35714286 -0.34285714 -0.32857143 -0.31428571 -0.3 -0.28571429 -0.27142857 -0.25714286 -0.24285714 -0.22857143 -0.21428571 -0.2 -0.18571429 -0.17142857 -0.15714286 -0.14285714 -0.12857143 -0.11428571 -0.1 -0.08571429 -0.07142857 -0.05714286 -0.04285714 -0.02857143 -0.01428571 0 0 0 0 0 0
  line L33 (-24.7944, -43.3762) -> (-24.449, -43.1996)
  arc A67 (-24.3149, -43.2424) -> (-24.449, -43.1996) centre (-24.4035, -43.2886) ccw
  arc A68 (-24.3149, -43.2424) -> (-23.7979, -44.1384) centre (-13.5, -37.5997) ccw
  arc A69 (-23.828, -44.276) -> (-23.7979, -44.1384) centre (-23.8823, -44.192) ccw
  line L34 (-23.828, -44.276) -> (-24.1538, -44.4865)
  spline S34 degree 5 poles (-24.1538, -44.4865) (-24.1585, -44.4896) (-24.1679, -44.4959) (-24.1818, -44.5056) (-24.1999, -44.5192) (-24.2218, -44.5371) (-24.2432, -44.5557) (-24.2644, -44.5747) (-24.2854, -44.594) (-24.3063, -44.6133) (-24.3271, -44.6329) (-24.3478, -44.6526) (-24.3683, -44.6726) (-24.3885, -44.6929) (-24.4085, -44.7135) (-24.4283, -44.7344) (-24.4479, -44.7556) (-24.4674, -44.777) (-24.4867, -44.7985) (-24.5059, -44.8202) (-24.525, -44.8421) (-24.5439, -44.8641) (-24.5627, -44.8864) (-24.5813, -44.9088) (-24.5998, -44.9314) (-24.6181, -44.9542) (-24.6363, -44.9772) (-24.6544, -45.0003) (-24.6723, -45.0236) (-24.6901, -45.0471) (-24.7078, -45.0707) (-24.7254, -45.0944) (-24.7428, -45.1183) (-24.7602, -45.1423) (-24.7773, -45.1665) (-24.7944, -45.1908) (-24.8113, -45.2153) (-24.8282, -45.2399) (-24.8449, -45.2647) (-24.8615, -45.2895) (-24.8779, -45.3145) (-24.8943, -45.3397) (-24.9105, -45.365) (-24.9266, -45.3904) (-24.9426, -45.4159) (-24.9585, -45.4415) (-24.9743, -45.4673) (-24.99, -45.4932) (-25.0055, -45.5192) (-25.021, -45.5453) (-25.0363, -45.5716) (-25.0515, -45.598) (-25.0666, -45.6245) (-25.0816, -45.651) (-25.0965, -45.6778) (-25.1113, -45.7046) (-25.1259, -45.7315) (-25.1405, -45.7586) (-25.1549, -45.7857) (-25.1693, -45.813) (-25.1835, -45.8403) (-25.1976, -45.8678) (-25.2116, -45.8954) (-25.2255, -45.9231) (-25.2393, -45.9509) (-25.253, -45.9787) (-25.2666, -46.0067) (-25.2801, -46.0348) (-25.2935, -46.063) (-25.3067, -46.0913) (-25.3199, -46.1197) (-25.3303, -46.1425) (-25.3381, -46.1596) (-25.3433, -46.171) (-25.3459, -46.1768) knots 0 0 0 0 0 0 0.01428571 0.02857143 0.04285714 0.05714286 0.07142857 0.08571429 0.1 0.11428571 0.12857143 0.14285714 0.15714286 0.17142857 0.18571429 0.2 0.21428571 0.22857143 0.24285714 0.25714286 0.27142857 0.28571429 0.3 0.31428571 0.32857143 0.34285714 0.35714286 0.37142857 0.38571429 0.4 0.41428571 0.42857143 0.44285714 0.45714286 0.47142857 0.48571429 0.5 0.51428571 0.52857143 0.54285714 0.55714286 0.57142857 0.58571429 0.6 0.61428571 0.62857143 0.64285714 0.65714286 0.67142857 0.68571429 0.7 0.71428571 0.72857143 0.74285714 0.75714286 0.77142857 0.78571429 0.8 0.81428571 0.82857143 0.84285714 0.85714286 0.87142857 0.88571429 0.9 0.91428571 0.92857143 0.94285714 0.95714286 0.97142857 0.98571429 1 1 1 1 1 1
  arc A70 (-25.3459, -46.1768) -> (-24.8561, -46.8155) centre (-13.5, -37.5997) ccw
  spline S35 degree 5 poles (-24.8561, -46.8155) (-24.8499, -46.8145) (-24.8375, -46.8124) (-24.8189, -46.8094) (-24.7942, -46.8052) (-24.7634, -46.7998) (-24.7326, -46.7944) (-24.7019, -46.7888) (-24.6713, -46.783) (-24.6408, -46.7772) (-24.6103, -46.7712) (-24.5799, -46.7651) (-24.5495, -46.7588) (-24.5192, -46.7524) (-24.489, -46.7459) (-24.4589, -46.7393) (-24.4289, -46.7325) (-24.3989, -46.7256) (-24.369, -46.7185) (-24.3392, -46.7114) (-24.3095, -46.7041) (-24.2798, -46.6966) (-24.2502, -46.689) (-24.2207, -46.6813) (-24.1913, -46.6735) (-24.162, -46.6655) (-24.1327, -46.6573) (-24.1036, -46.6491) (-24.0745, -46.6406) (-24.0455, -46.6321) (-24.0166, -46.6234) (-23.9878, -46.6146) (-23.9591, -46.6056) (-23.9305, -46.5965) (-23.902, -46.5872) (-23.8736, -46.5778) (-23.8452, -46.5682) (-23.817, -46.5585) (-23.7889, -46.5486) (-23.7608, -46.5386) (-23.7329, -46.5284) (-23.7051, -46.5181) (-23.6774, -46.5076) (-23.6498, -46.497) (-23.6223, -46.4862) (-23.595, -46.4752) (-23.5677, -46.4641) (-23.5405, -46.4528) (-23.5135, -46.4413) (-23.4866, -46.4297) (-23.4598, -46.4179) (-23.4332, -46.4059) (-23.4067, -46.3938) (-23.3804, -46.3814) (-23.3542, -46.3688) (-23.3281, -46.3561) (-23.3021, -46.3432) (-23.2763, -46.3301) (-23.2506, -46.3169) (-23.2251, -46.3034) (-23.1998, -46.2897) (-23.1747, -46.2757) (-23.1498, -46.2615) (-23.1252, -46.2469) (-23.1008, -46.232) (-23.0765, -46.217) (-23.0524, -46.2018) (-23.0284, -46.1865) (-23.0045, -46.171) (-22.981, -46.1551) (-22.958, -46.1386) (-22.9402, -46.1247) (-22.9272, -46.1138) (-22.9187, -46.1064) (-22.9145, -46.1026) knots -1 -1 -1 -1 -1 -1 -0.98571429 -0.97142857 -0.95714286 -0.94285714 -0.92857143 -0.91428571 -0.9 -0.88571429 -0.87142857 -0.85714286 -0.84285714 -0.82857143 -0.81428571 -0.8 -0.78571429 -0.77142857 -0.75714286 -0.74285714 -0.72857143 -0.71428571 -0.7 -0.68571429 -0.67142857 -0.65714286 -0.64285714 -0.62857143 -0.61428571 -0.6 -0.58571429 -0.57142857 -0.55714286 -0.54285714 -0.52857143 -0.51428571 -0.5 -0.48571429 -0.47142857 -0.45714286 -0.44285714 -0.42857143 -0.41428571 -0.4 -0.38571429 -0.37142857 -0.35714286 -0.34285714 -0.32857143 -0.31428571 -0.3 -0.28571429 -0.27142857 -0.25714286 -0.24285714 -0.22857143 -0.21428571 -0.2 -0.18571429 -0.17142857 -0.15714286 -0.14285714 -0.12857143 -0.11428571 -0.1 -0.08571429 -0.07142857 -0.05714286 -0.04285714 -0.02857143 -0.01428571 0 0 0 0 0 0
  line L35 (-22.9145, -46.1026) -> (-22.6266, -45.8426)
  arc A71 (-22.4859, -45.8492) -> (-22.6266, -45.8426) centre (-22.5596, -45.9168) ccw
  arc A72 (-22.4859, -45.8492) -> (-21.7547, -46.5809) centre (-13.5, -37.5997) ccw
  arc A73 (-21.7482, -46.7216) -> (-21.7547, -46.5809) centre (-21.8223, -46.6545) ccw
  line L36 (-21.7482, -46.7216) -> (-22.0083, -47.0093)
  spline S36 degree 5 poles (-22.0083, -47.0093) (-22.0121, -47.0135) (-22.0196, -47.0219) (-22.0305, -47.0349) (-22.0444, -47.0528) (-22.0609, -47.0758) (-22.0768, -47.0993) (-22.0923, -47.1231) (-22.1076, -47.1471) (-22.1228, -47.1712) (-22.1379, -47.1955) (-22.1527, -47.2199) (-22.1673, -47.2445) (-22.1816, -47.2694) (-22.1956, -47.2945) (-22.2094, -47.3198) (-22.2228, -47.3453) (-22.2361, -47.371) (-22.2492, -47.3968) (-22.2621, -47.4227) (-22.2748, -47.4488) (-22.2874, -47.475) (-22.2998, -47.5013) (-22.312, -47.5278) (-22.324, -47.5544) (-22.3358, -47.5812) (-22.3474, -47.6081) (-22.3589, -47.6351) (-22.3702, -47.6623) (-22.3813, -47.6895) (-22.3923, -47.7169) (-22.4031, -47.7444) (-22.4138, -47.772) (-22.4243, -47.7997) (-22.4346, -47.8275) (-22.4448, -47.8554) (-22.4549, -47.8834) (-22.4647, -47.9115) (-22.4745, -47.9398) (-22.4841, -47.9681) (-22.4935, -47.9965) (-22.5028, -48.025) (-22.5119, -48.0536) (-22.5209, -48.0823) (-22.5298, -48.1111) (-22.5385, -48.14) (-22.5471, -48.169) (-22.5555, -48.1981) (-22.5638, -48.2272) (-22.5719, -48.2565) (-22.5799, -48.2858) (-22.5878, -48.3152) (-22.5955, -48.3447) (-22.6031, -48.3742) (-22.6106, -48.4039) (-22.6179, -48.4336) (-22.6251, -48.4634) (-22.6322, -48.4933) (-22.6391, -48.5233) (-22.6459, -48.5533) (-22.6526, -48.5835) (-22.6591, -48.6137) (-22.6655, -48.6439) (-22.6718, -48.6743) (-22.6779, -48.7047) (-22.6839, -48.7351) (-22.6898, -48.7657) (-22.6955, -48.7963) (-22.7012, -48.827) (-22.7067, -48.8578) (-22.712, -48.8886) (-22.7162, -48.9133) (-22.7193, -48.9319) (-22.7213, -48.9443) (-22.7223, -48.9504) knots 0 0 0 0 0 0 0.01428571 0.02857143 0.04285714 0.05714286 0.07142857 0.08571429 0.1 0.11428571 0.12857143 0.14285714 0.15714286 0.17142857 0.18571429 0.2 0.21428571 0.22857143 0.24285714 0.25714286 0.27142857 0.28571429 0.3 0.31428571 0.32857143 0.34285714 0.35714286 0.37142857 0.38571429 0.4 0.41428571 0.42857143 0.44285714 0.45714286 0.47142857 0.48571429 0.5 0.51428571 0.52857143 0.54285714 0.55714286 0.57142857 0.58571429 0.6 0.61428571 0.62857143 0.64285714 0.65714286 0.67142857 0.68571429 0.7 0.71428571 0.72857143 0.74285714 0.75714286 0.77142857 0.78571429 0.8 0.81428571 0.82857143 0.84285714 0.85714286 0.87142857 0.88571429 0.9 0.91428571 0.92857143 0.94285714 0.95714286 0.97142857 0.98571429 1 1 1 1 1 1
  arc A74 (-22.7223, -48.9504) -> (-22.0839, -49.4406) centre (-13.5, -37.5997) ccw
  spline S37 degree 5 poles (-22.0839, -49.4406) (-22.0782, -49.438) (-22.0667, -49.4329) (-22.0496, -49.4251) (-22.0268, -49.4147) (-21.9984, -49.4015) (-21.9701, -49.3883) (-21.9419, -49.3749) (-21.9138, -49.3615) (-21.8858, -49.3479) (-21.8579, -49.3342) (-21.8302, -49.3204) (-21.8025, -49.3065) (-21.7749, -49.2925) (-21.7474, -49.2784) (-21.72, -49.2642) (-21.6928, -49.2499) (-21.6656, -49.2355) (-21.6385, -49.2209) (-21.6116, -49.2063) (-21.5848, -49.1915) (-21.558, -49.1767) (-21.5314, -49.1617) (-21.5049, -49.1466) (-21.4786, -49.1314) (-21.4523, -49.1161) (-21.4262, -49.1007) (-21.4001, -49.0851) (-21.3742, -49.0695) (-21.3485, -49.0537) (-21.3228, -49.0378) (-21.2973, -49.0218) (-21.2719, -49.0057) (-21.2466, -48.9895) (-21.2214, -48.9732) (-21.1964, -48.9567) (-21.1715, -48.9401) (-21.1468, -48.9235) (-21.1221, -48.9066) (-21.0977, -48.8897) (-21.0733, -48.8727) (-21.0491, -48.8555) (-21.0251, -48.8382) (-21.0012, -48.8208) (-20.9774, -48.8032) (-20.9538, -48.7855) (-20.9304, -48.7677) (-20.9071, -48.7498) (-20.8839, -48.7318) (-20.861, -48.7136) (-20.8381, -48.6953) (-20.8155, -48.6768) (-20.7931, -48.6582) (-20.7708, -48.6394) (-20.7488, -48.6205) (-20.7269, -48.6014) (-20.7052, -48.5823) (-20.6836, -48.563) (-20.6622, -48.5435) (-20.6411, -48.5239) (-20.6201, -48.5041) (-20.5995, -48.4841) (-20.5792, -48.4639) (-20.5592, -48.4434) (-20.5394, -48.4228) (-20.5199, -48.402) (-20.5005, -48.3811) (-20.4813, -48.3601) (-20.4622, -48.3389) (-20.4436, -48.3175) (-20.4257, -48.2956) (-20.4121, -48.2775) (-20.4023, -48.2637) (-20.3961, -48.2542) (-20.393, -48.2495) knots -1 -1 -1 -1 -1 -1 -0.98571429 -0.97142857 -0.95714286 -0.94285714 -0.92857143 -0.91428571 -0.9 -0.88571429 -0.87142857 -0.85714286 -0.84285714 -0.82857143 -0.81428571 -0.8 -0.78571429 -0.77142857 -0.75714286 -0.74285714 -0.72857143 -0.71428571 -0.7 -0.68571429 -0.67142857 -0.65714286 -0.64285714 -0.62857143 -0.61428571 -0.6 -0.58571429 -0.57142857 -0.55714286 -0.54285714 -0.52857143 -0.51428571 -0.5 -0.48571429 -0.47142857 -0.45714286 -0.44285714 -0.42857143 -0.41428571 -0.4 -0.38571429 -0.37142857 -0.35714286 -0.34285714 -0.32857143 -0.31428571 -0.3 -0.28571429 -0.27142857 -0.25714286 -0.24285714 -0.22857143 -0.21428571 -0.2 -0.18571429 -0.17142857 -0.15714286 -0.14285714 -0.12857143 -0.11428571 -0.1 -0.08571429 -0.07142857 -0.05714286 -0.04285714 -0.02857143 -0.01428571 0 0 0 0 0 0
  line L37 (-20.393, -48.2495) -> (-20.1822, -47.9239)
  arc A75 (-20.0446, -47.8938) -> (-20.1822, -47.9239) centre (-20.0983, -47.9782) ccw
  arc A76 (-20.0446, -47.8938) -> (-19.1489, -48.4113) centre (-13.5, -37.5997) ccw
  arc A77 (-19.1062, -48.5455) -> (-19.1489, -48.4113) centre (-19.1952, -48.4999) ccw
  line L38 (-19.1062, -48.5455) -> (-19.283, -48.8907)